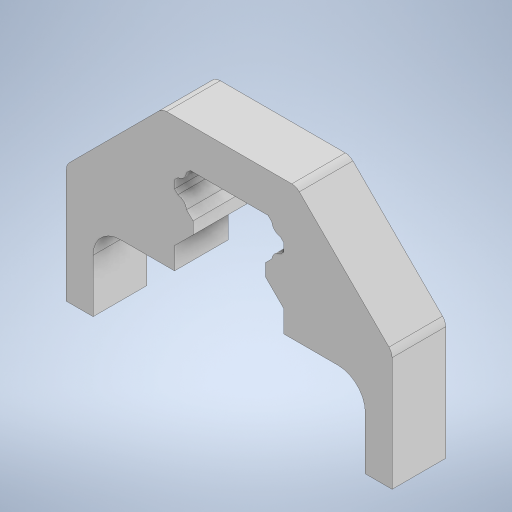
# Autodesk Inventor part: Spacermount
Saved by Autodesk Inventor 2023 (Build 270158000, 158)
## iProperties
Created: 2022-07-28
Part Number: Spacermount
Material: Generic
Document SubType Name: Modeling
Designer: plebbb
Density: 1 g/cm^3
Appearance: Default
Author: plebbb
Autodesk Inventor part; units mm, degrees
ref_plane "YZ Plane" through (0, 0, 0) normal (1, 0, 0) x (0, 1, 0)
ref_plane "XZ Plane" through (0, 0, 0) normal (0, 1, 0) x (-1, 0, 0)
ref_plane "XY Plane" through (0, 0, 0) normal (0, 0, 1) x (1, 0, 0)
sketch "Sketch1" plane through (0, 0, 0) normal (0, 0, 1) x (1, 0, 0)
  line L0 (10.08, 0) -> (50.72, 0)
  line L1 (60.8, 0) -> (60.8, 25)
  line L2 (60.8, 25) -> (0, 25)
  line L3 (0, 25) -> (0, 0)
  line L4 (0, 0) -> (0, -15)
  line L5 (0, -15) -> (5, -15)
  line L6 (5, -15) -> (5, -5.08)
  line L7 (55.8, -5.08) -> (55.8, -15)
  line L8 (55.8, -15) -> (60.8, -15)
  line L9 (60.8, -15) -> (60.8, 0)
  arc A0 (10.08, 0) -> (5, -5.08) centre (10.08, -5.08) ccw
  arc A1 (55.8, -5.08) -> (50.72, 0) centre (50.72, -5.08) ccw
  line L10 (0, 7.1) -> (17.9, 25)
  line L11 (42.9, 25) -> (60.8, 7.1)
  point P0 (55.8, -10.04)
  point P1 (5, -10.04)
  dimension "d17" = 25
  dimension "d18" = 60.8
  dimension "d19" = 50.8
  dimension "d20" = 15
  dimension "d21" = 5.08
  dimension "d22" = 25
  dimension "d23" = 45
  constraints: 24 end point, 6 point on line, 4 perpendicular, 4 point on circle, 4 tangent, 3 equal length, 3 vertical, 2 centre point, 2 midpoint, 2 parallel, 1 equal radius, 1 horizontal, 1 horizontal alignment
  measures "d17" distance of L1.start L1.end
  measures "d18" distance of L1.end L2.end
  measures "d19" distance of point (55.8, -10.04) point (5, -10.04)
  measures "d20" distance of L3.end L4.end
  measures "d21" radius of A0
  measures "d22" distance of L11.start L10.end
  measures "d23" angle of L2 L10
extrude "Extrusion1" add sketch "Sketch1" along normal blind 10 contours A0 L6 L5 L4 L3 L10 L2 L11 L1 L9 L8 L7 A1 L0
sketch "Sketch2" plane through (-9.4958, -11.5954, 10) normal (0, 0, 1) x (1, 0, 0)
  line L0 (39.8958, 11.5954) -> (48.8958, 11.5954)
  line L1 (48.8958, 11.5954) -> (49.8958, 12.5954)
  line L2 (49.8958, 12.5954) -> (49.8958, 15.5954)
  line L3 (46.4458, 19.0454) -> (46.4458, 21.4721)
  line L4 (49.8958, 15.5954) -> (46.4458, 19.0454)
  line L5 (49.8958, 12.5954) -> (49.8958, 11.5954)
  line L6 (48.8958, 11.5954) -> (49.8958, 11.5954)
  line L7 (39.8958, 11.5954) -> (30.8958, 11.5954)
  line L8 (30.8958, 11.5954) -> (29.8958, 12.5954)
  line L9 (29.8958, 11.5954) -> (30.8958, 11.5954)
  line L10 (29.8958, 15.5954) -> (33.3458, 19.0454)
  line L11 (30.4166, 24.4012) -> (29.8958, 24.9221)
  line L12 (29.8958, 24.9221) -> (29.8958, 26.2554)
  line L13 (33.3458, 19.0454) -> (33.3458, 21.4721)
  line L14 (29.8958, 26.2554) -> (30.4166, 26.7762)
  line L15 (32.1286, 22.6893) -> (30.4166, 24.4012) construction
  arc A0 (32.1286, 22.6893) -> (30.4166, 24.4012) centre (30.1469, 22.4195) ccw
  line L16 (33.3458, 21.4721) -> (32.1286, 22.6893)
  line L17 (32.1286, 28.4882) -> (30.4166, 26.7762) construction
  arc A1 (30.4166, 26.7762) -> (32.1286, 28.4882) centre (30.1469, 28.758) ccw
  line L18 (32.1286, 28.4882) -> (32.7358, 29.0954)
  line L19 (32.7358, 29.0954) -> (39.8958, 29.0954)
  line L20 (39.8958, 29.0954) -> (39.8958, 11.5954) construction
  line L21 (29.8958, 12.5954) -> (29.8958, 11.5954)
  line L22 (29.8958, 12.5954) -> (29.8958, 15.5954)
  line L23 (46.4458, 21.4721) -> (47.663, 22.6893)
  line L24 (47.663, 22.6893) -> (49.375, 24.4012) construction
  arc A2 (49.375, 24.4012) -> (47.663, 22.6893) centre (49.6447, 22.4195) ccw
  line L25 (49.375, 24.4012) -> (49.8958, 24.9221)
  line L26 (49.8958, 24.9221) -> (49.8958, 26.2554)
  line L27 (49.8958, 26.2554) -> (49.375, 26.7762)
  line L28 (47.0558, 29.0954) -> (39.8958, 29.0954)
  line L29 (47.663, 28.4882) -> (49.375, 26.7762) construction
  arc A3 (47.663, 28.4882) -> (49.375, 26.7762) centre (49.6447, 28.758) ccw
  line L30 (47.663, 28.4882) -> (47.0558, 29.0954)
  line L31 (70.2958, -3.4046) -> (70.2958, 18.6954) projected
  line L32 (52.3958, 36.5954) -> (27.3958, 36.5954) projected
  line L33 (9.4958, 18.6954) -> (9.4958, -3.4046) projected
  line L34 (19.5758, 11.5954) -> (60.2158, 11.5954) projected
  line L35 (65.2958, -3.4046) -> (70.2958, -3.4046) projected
  line L36 (9.4958, -3.4046) -> (14.4958, -3.4046) projected
  line L37 (14.4958, -3.4046) -> (14.4958, 6.5154) projected
  arc A4 (19.5758, 11.5954) -> (14.4958, 6.5154) centre (19.5758, 6.5154) ccw projected
  arc A5 (65.2958, 6.5154) -> (60.2158, 11.5954) centre (60.2158, 6.5154) ccw projected
  line L38 (65.2958, 6.5154) -> (65.2958, -3.4046) projected
  line L39 (70.2958, 18.6954) -> (52.3958, 36.5954) projected
  line L40 (27.3958, 36.5954) -> (9.4958, 18.6954) projected
  point P0 (52.225, 35.4)
  point P1 (49.8958, 14.0954)
  point P2 (14.4958, -3.175)
  point P3 (0, 11.5954)
  point P4 (29.8958, 12.0954)
  point P5 (39.8958, 36.5954)
  dimension "d13" = 1
  dimension "d11" = 3
  dimension "d9" = 135
  dimension "d3" = 2
  dimension "d10" = 3.45
  dimension "d8" = 17.5
  dimension "d4" = 7.16
  dimension "d5" = 2.375
  dimension "d6" = 1.3333
  dimension "d7" = 2.4211
  dimension "d12" = 10
  dimension "d2" = 15.4
  constraints: 62 end point, 14 symmetric about line, 8 point on circle, 6 perpendicular, 4 centre point, 4 collinear, 4 vertical alignment, 3 midpoint, 2 horizontal, 2 parallel, 2 vertical, 1 equal radius, 1 horizontal alignment, 2 other
  measures "d13" distance from line of L0 L1.end
  measures "d11" distance of L1.end L2.end
  measures "d9" angle of L2 L4
  measures "d3" radius of A3
  measures "d10" horizontal distance of L3.start L2.end
  measures "d8" distance of L19.end L0.start
  measures "d4" distance of L28.start L19.end
  measures "d5" distance of L24.end L27.end
  measures "d6" distance of L25.end L26.end
  measures "d7" distance of L23.end L24.end
  measures "d12" horizontal distance of L0.start L1.end
  measures "d2" horizontal distance of point (14.496, -3.175) point (29.896, 12.095)
extrude "Extrusion2" cut sketch "Sketch2" against normal up to surface (10 mm away) contours L7 L8 L22 L10 L13 L16 A0 L11 L12 L14 A1 L18 L19 L28 L30 A3 L27 L26 L25 A2 L23 L3 L4 L2 L1 L0 | L1 L5 L6 | L9 L21 L8
fillet "Fillet1" radius 2 4 edges at (0, 7.1, 5) (17.9, 25, 5) (42.9, 25, 5) (60.8, 7.1, 5)
thicken "Thicken1" operation cut thickness 0.2 both sides no extend neighbours no toward (-1, 0, 0) faces at (20.4, 2.6667, 6.6667) (22.7, 6.3, 6.6667) (23.85, 9.0678, 6.6667) (23.0385, 10.6881, 6.6667) (21.6037, 12.5827, 3.3333) (20.5736, 13.1531, 6.6667) (20.4, 14.2156, 6.6667) (20.7472, 15.0072, 6.6667) (21.4743, 15.3398, 3.3333) (23.0376, 17.2976, 6.6667) (32.7867, 17.5, 6.6667) (37.9648, 17.0952, 6.6667) (38.2267, 16.6103, 3.3333) (40.2264, 14.8336, 3.3333) (40.4, 13.7711, 6.6667) (40.0528, 12.9794, 6.6667) (39.7368, 12.7812, 3.3333) (37.3557, 10.2824, 6.6667) (36.95, 8.2589, 6.6667) (39.25, 5.15, 6.6667) (40.4, 1.3333, 6.6667)
body "Solid1"
